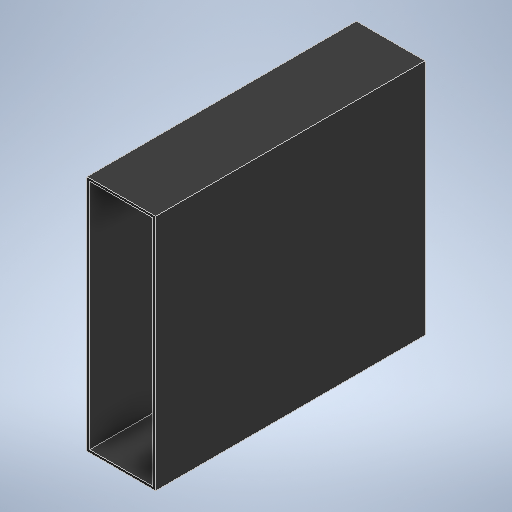
# Autodesk Inventor part: Tube_Of_Underlayment_For_Joist_With_Length_6.5_Inches
Saved by Autodesk Inventor 2025 (Build 290162010, 162A)
## iProperties
Created: 2024-09-15
Part Number: Tube_Of_Underlayment_For_Joist_With_Length_6.5_Inches
Material: Rubber
Document SubType Name: Modeling
Designer: Tom
Density: 0.93 g/cm^3
Appearance: Rubber - Black
Author: Tom
Autodesk Inventor part; units mm, degrees
ref_plane "YZ Plane" through (0, 0, 0) normal (1, 0, 0) x (0, 1, 0)
ref_plane "XZ Plane" through (0, 0, 0) normal (0, 1, 0) x (-1, 0, 0)
ref_plane "XY Plane" through (0, 0, 0) normal (0, 0, 1) x (1, 0, 0)
sketch "Sketch1" plane through (0, 0, 0) normal (0, 0, 1) x (1, 0, 0)
  line L0 (0, 0) -> (38.1, 0)
  line L1 (38.1, 0) -> (38.1, 139.7)
  line L2 (38.1, 139.7) -> (0, 139.7)
  line L3 (0, 139.7) -> (0, 0)
  line L4 (-1.5875, 141.2875) -> (39.6875, 141.2875)
  line L5 (39.6875, 141.2875) -> (39.6875, -1.5875)
  line L6 (39.6875, -1.5875) -> (-1.5875, -1.5875)
  line L7 (-1.5875, -1.5875) -> (-1.5875, 141.2875)
  dimension "d1" = 139.7
  dimension "d2" = 38.1
  dimension "d3" = 1.5875
  constraints: 16 end point, 4 parallel, 2 perpendicular, 1 horizontal, 3 other
  measures "d1" distance of L2.end L0.start
  measures "d2" distance of L0.start L0.end
  measures "d3" distance between parallel lines of L5 L1
extrude "Extrusion1" add sketch "Sketch1" along normal blind 161.925
body "Solid1"
